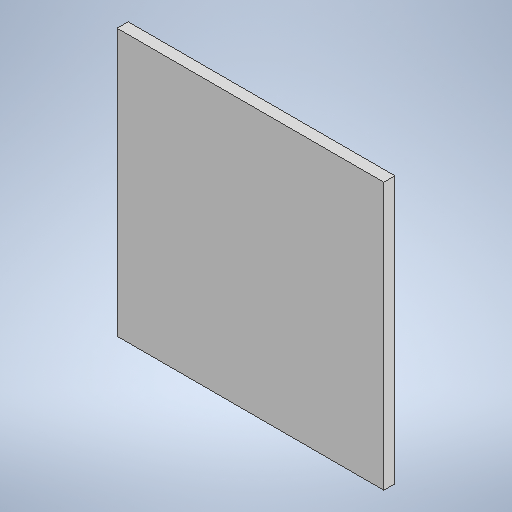
# Autodesk Inventor part: bread
Saved by Autodesk Inventor 2025.1 (Build 291241020, 241B)
## iProperties
Created: 2024-10-30
Part Number: bread
Material: Generic
Document SubType Name: Modeling
Designer: jjk
Density: 1 g/cm^3
Appearance: Default
Author: jjk
Autodesk Inventor part; units mm, degrees
ref_plane "YZ Plane" through (0, 0, 0) normal (1, 0, 0) x (0, 1, 0)
ref_plane "XZ Plane" through (0, 0, 0) normal (0, 1, 0) x (-1, 0, 0)
ref_plane "XY Plane" through (0, 0, 0) normal (0, 0, 1) x (1, 0, 0)
sketch "Sketch1" plane through (0, 0, 0) normal (0, 0, 1) x (1, 0, 0)
  line L0 (157.4321, 276.7642) -> (309.8321, 276.7642)
  line L1 (309.8321, 276.7642) -> (309.8321, 124.3642)
  line L2 (309.8321, 124.3642) -> (157.4321, 124.3642)
  line L3 (157.4321, 124.3642) -> (157.4321, 276.7642)
  point P0 (0, 0)
  dimension "d0" = 152.4
  dimension "d1" = 152.4
  constraints: 8 end point, 2 parallel, 1 horizontal, 1 perpendicular
  measures "d0" distance of L2.end L0.start
  measures "d1" distance of L1.end L2.end
extrude "Extrusion1" add sketch "Sketch1" along normal blind 6.35
body "Solid1"
